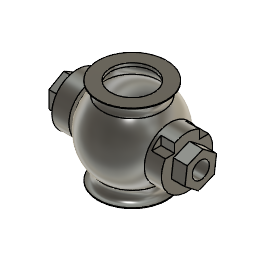
Underneath Whistle (Ball Part) (Autodesk Fusion 360 design; units mm, degrees)
part number: 2026-04-10-14-00-23-063
Autodesk Fusion 360 part; units mm, degrees
note: some values were not read from the file. Set by a fixed rule: which sketch regions a step uses.
sketch "Sketch1" plane through (0, 0, 0) normal (1, 0, 0) x (0, 1, 0)
  line L0 (0, 63.5) -> (25.4, 63.5)
  arc A0 (25.4, 63.5) -> (21.8966, 54.7414) centre (25.4, 58.42) ccw
  line L1 (0, 0) -> (25.4, 0)
  arc A1 (21.8966, 8.7586) -> (25.4, 0) centre (25.4, 5.08) ccw
  line L2 (0, 61.595) -> (19.1783, 61.595)
  line L3 (0, 1.905) -> (19.1783, 1.905)
  arc A2 (20.5828, 10.1381) -> (20.5828, 53.3619) centre (0, 31.75) ccw
  line L4 (0, 63.5) -> (0, 61.595)
  line L5 (0, 1.905) -> (0, 0)
  arc A3 (20.5828, 10.1381) -> (19.1783, 1.905) centre (25.4, 5.08) ccw
  arc A4 (21.8966, 8.7586) -> (21.8966, 54.7414) centre (0, 31.75) ccw
  arc A5 (19.1783, 61.595) -> (20.5828, 53.3619) centre (25.4, 58.42) ccw
  dimension "d1" = 25.4
  dimension "d3" = 10.16
  dimension "d4" = 10.16
  dimension "d5" = 25.4
  dimension "d10" = 13.97
  dimension "d11" = 59.69
  dimension "d12" = 13.97
  constraint horizontal L0
  constraint tangent L0 A0
  constraint tangent A0 A4
  constraint coincident L1.start L5.end
  constraint horizontal L1
  constraint tangent A1 A4
  constraint tangent L1 A1
  constraint perpendicular L1 L5
  constraint concentric A0 A5
  constraint concentric A2 A4
  constraint tangent L2 A2
  constraint concentric A1 A3
  constraint tangent L3 A2
  constraint collinear L4 L5
  measures "d1" distance of L0.start L0.end
  measures "d3" diameter of A0
  measures "d4" diameter of A1
  measures "d5" distance of L1.start L1.end
  measures "d10" diameter of A5
  measures "d11" diameter of A2
  measures "d12" diameter of A3
revolve "Revolve1" add sketch "Sketch1" angle 360 about axis through (0, 0, 1.75) along (0, 0, 1)
extrude "Extrude1" add 1 faces at (4.958, 9.5122, 63.5) along direction (0, 0, 1) blind 0.508
extrude "Extrude2" add 1 faces at (4.958, 9.5122, 0) along direction (0, 0, -1) blind 0.508
ref_plane "WorkPlane1" through (0, 27.94, 0) normal (0, 1, 0) x (0, 0, 1)
sketch "Sketch3" plane through (0, 27.94, 0) normal (0, 1, 0) x (1, 0, 0)
  line L0 (0, 0) -> (0, -31.75)
  circle A0 centre (0, -31.75) radius 15.0749
  circle A1 centre (0, -31.75) radius 19.05
  dimension "d19" = 31.75
  dimension "d20" = 38.1
  constraint coincident L0.start origin
  constraint vertical L0
  constraint coincident L0.end A0.centre
  constraint concentric A0 A1
  measures "d19" distance of L0.start L0.end
  measures "d20" diameter of A1
extrude "Extrude3" add sketch "Sketch3" along normal blind 12.7 contours A0 | A1
sketch "Sketch4" plane through (0, 40.64, 0) normal (0, 1, 0) x (-1, 0, 0)
  circle A0 centre (0, 31.75) radius 19.05
  circle A1 centre (0, 31.75) radius 12.7
  dimension "d23" = 25.4
  constraint concentric A0 A1
  measures "d23" diameter of A1
extrude "Extrude4" cut sketch "Sketch4" against normal blind 25.4 contours A1
sketch "Sketch5" plane through (0, 0, -0.508) normal (0, 0, -1) x (1, 0, 0)
  circle A0 centre (0, 0) radius 25.4
  circle A1 centre (0, 0) radius 15.875
  dimension "d26" = 31.75
  constraint coincident A0.centre A1.centre
  measures "d26" diameter of A1
extrude "Extrude5" cut sketch "Sketch5" against normal blind 7.62 contours A1
move_body "Move1" bodies 1 to x (0, -1, 0) y (1, 0, 0) z (0, 0, 1) at (0, 0, 0)
sketch "Sketch6" plane through (0, 0, 64.008) normal (0, 0, 1) x (-1, 0, 0)
  circle A0 centre (0, 0) radius 25.4
sketch "Sketch7" plane through (0, 0, 64.008) normal (0, 0, 1) x (-1, 0, 0)
  circle A0 centre (0, 0) radius 15.875
  dimension "d30" = 31.75
  constraint coincident A0.centre origin
  measures "d30" diameter of A0
extrude "Extrude6" cut sketch "Sketch7" against normal blind 7.62
ref_plane "WorkPlane2" through (-27.94, 0, 0) normal (1, 0, 0) x (0, 1, 0)
sketch "Sketch8" plane through (-27.94, 0, 0) normal (1, 0, 0) x (0, 1, 0)
  line L0 (0, 0) -> (0, 31.75)
  circle A0 centre (0, 31.75) radius 15.0749
  circle A1 centre (0, 31.75) radius 19.05
  dimension "d34" = 31.75
  dimension "d35" = 38.1
  constraint coincident L0.start origin
  constraint vertical L0
  constraint coincident L0.end A0.centre
  constraint concentric A0 A1
  measures "d34" distance of L0.start L0.end
  measures "d35" diameter of A1
extrude "Extrude7" add sketch "Sketch8" against normal blind 12.7 contours A0 | A1
sketch "Sketch9" plane through (-40.64, 0, 0) normal (-1, 0, 0) x (0, -1, 0)
  circle A0 centre (0, 31.75) radius 19.05
  circle A1 centre (0, 31.75) radius 7.9375
  dimension "d39" = 15.875
  constraint concentric A0 A1
  measures "d39" diameter of A1
extrude "Extrude8" cut sketch "Sketch9" against normal blind 20.32 contours A1
sketch "Sketch10" plane through (-40.64, 0, 0) normal (-1, 0, 0) x (0, -1, 0)
  circle A0 centre (0, 31.75) radius 7.9375
  circle A1 centre (0, 31.75) radius 19.05
  line L0 (0, 44.45) -> (-10.9985, 38.1)
  line L1 (-10.9985, 38.1) -> (-10.9985, 25.4)
  line L2 (-10.9985, 25.4) -> (0, 19.05)
  line L3 (0, 19.05) -> (10.9985, 25.4)
  line L4 (10.9985, 25.4) -> (10.9985, 38.1)
  line L5 (10.9985, 38.1) -> (0, 44.45)
  point P0 (0, 31.75)
  dimension "d42" = 12.7
  constraint coincident P0 A0.centre
  measures "d42" distance of L0.start P0
extrude "Extrude9" add sketch "Sketch10" along normal blind 10.16 contours A0 | L0 L1 L2 L3 L4 L5
sketch "Sketch11" plane through (-50.8, 0, 0) normal (-1, 0, 0) x (0, -1, 0)
  line L0 (10.9985, 38.1) -> (0, 44.45)
  line L1 (0, 44.45) -> (-10.9985, 38.1)
  line L2 (-10.9985, 38.1) -> (-10.9985, 25.4)
  line L3 (-10.9985, 25.4) -> (0, 19.05)
  line L4 (0, 19.05) -> (10.9985, 25.4)
  line L5 (10.9985, 25.4) -> (10.9985, 38.1)
  circle A0 centre (0, 31.75) radius 6.35
  dimension "d45" = 12.7
  measures "d45" diameter of A0
extrude "Extrude10" add sketch "Sketch11" along normal blind 6.35 contours A0
fillet "Fillet1" radius 6.35 1 edges at (-57.15, 5.9203, 29.4537)
sketch "Sketch12" plane through (40.64, 0, 0) normal (1, 0, 0) x (0, 1, 0)
  circle A0 centre (0, 31.75) radius 12.7
  circle A1 centre (0, 31.75) radius 19.05
  circle A2 centre (0, 31.75) radius 12.7
  circle A3 centre (0, 31.75) radius 6.35
  dimension "d50" = 12.7
  constraint concentric A0 A2
  constraint concentric A2 A3
  measures "d50" diameter of A3
extrude "Extrude11" add sketch "Sketch12" against normal blind 3.81 contours A0 A2
sketch "Sketch13" plane through (40.64, 0, 0) normal (1, 0, 0) x (0, 1, 0)
  circle A0 centre (0, 31.75) radius 6.35
  circle A1 centre (0, 31.75) radius 19.05
  line L0 (1.6803, 44.3384) -> (-10.0617, 39.4993)
  line L1 (-10.0617, 39.4993) -> (-11.742, 26.911)
  line L2 (-11.742, 26.911) -> (-1.6803, 19.1616)
  line L3 (-1.6803, 19.1616) -> (10.0617, 24.0007)
  line L4 (10.0617, 24.0007) -> (11.742, 36.589)
  line L5 (11.742, 36.589) -> (1.6803, 44.3384)
  point P0 (0, 31.75)
  dimension "d53" = 12.7
  constraint coincident P0 A0.centre
  measures "d53" distance of L0.start P0
extrude "Extrude12" add sketch "Sketch13" along normal blind 10.16 contours L0 L1 L2 L3 L4 L5
ref_plane "WorkPlane3" through (0, 0, 41.91) normal (0, 0, 1) x (1, 0, 0)
sketch "Sketch14" plane through (0, 0, 41.91) normal (0, 0, 1) x (1, 0, 0)
  line L0 (33.02, 9.1745) -> (33.02, -9.1643)
  line L1 (30.48, -9.1643) -> (40.64, -9.1643)
  line L2 (40.64, -9.1643) -> (40.64, -16.7843)
  line L3 (40.64, -16.7843) -> (30.48, -16.7843)
  line L4 (30.48, -16.7843) -> (30.48, -9.1643)
  line L5 (30.48, 9.1745) -> (40.64, 9.1745)
  line L6 (40.64, 9.1745) -> (40.64, 16.7945)
  line L7 (40.64, 16.7945) -> (30.48, 16.7945)
  line L8 (30.48, 16.7945) -> (30.48, 9.1745)
  point P0 (33.02, 0.0051)
  dimension "d57" = 18.3388
  dimension "d58" = 7.62
  dimension "d59" = 10.16
  dimension "d60" = 7.62
  dimension "d61" = 10.16
  constraint midpoint L0 P0
  constraint vertical L0
  constraint horizontal L1
  constraint vertical L2
  constraint horizontal L3
  constraint vertical L4
  constraint horizontal L5
  constraint vertical L6
  constraint horizontal L7
  constraint vertical L8
  measures "d57" distance of L0.start L0.end
  measures "d58" distance of L1.start L3.end
  measures "d59" distance of L2.end L3.end
  measures "d60" distance of L5.start L7.end
  measures "d61" distance of L6.end L7.end
extrude "Extrude13" cut sketch "Sketch14" along normal blind 12.7
